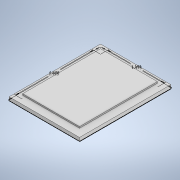
# Autodesk Inventor part: Valve Holder-3valve-withwirebox-lidforbox
Saved by Autodesk Inventor 2020 (Build 240168000, 168)
## iProperties
Created: 2022-02-08
Part Number: Valve Holder-3valve-withwirebox-lidforbox
Material: Generic
Document SubType Name: Modeling
Designer: Beaucage
Density: 1 g/cm^3
Appearance: Default
Author: Beaucage
Autodesk Inventor part; units mm, degrees
ref_plane "YZ Plane" through (0, 0, 0) normal (1, 0, 0) x (0, 1, 0)
ref_plane "XZ Plane" through (0, 0, 0) normal (0, 1, 0) x (-1, 0, 0)
ref_plane "XY Plane" through (0, 0, 0) normal (0, 0, 1) x (1, 0, 0)
sketch "Sketch1" plane through (0, 0, 0) normal (0, 1, 0) x (-1, 0, 0)
  line L0 (0, 0) -> (37.465, 0)
  line L1 (37.465, 0) -> (37.465, -48.641)
  line L2 (37.465, -48.641) -> (0, -48.641)
  line L3 (0, -48.641) -> (0, 0)
  line L4 (4.2291, -4.2291) -> (34.5059, -4.2291)
  line L5 (34.5059, -4.2291) -> (34.5059, -45.6819)
  line L6 (34.5059, -45.6819) -> (4.2291, -45.6819)
  line L7 (4.2291, -45.6819) -> (4.2291, -4.2291)
  line L8 (4.2291, -4.2291) -> (34.5059, -45.6819) construction
  line L9 (34.5059, -4.2291) -> (4.2291, -45.6819) construction
  point P0 (19.3675, -24.9555)
  dimension "d0" = 37.465
  dimension "d1" = 48.641
  dimension "d2" = 30.2768
  dimension "d3" = 41.4528
  constraints: 20 end point, 4 parallel, 2 horizontal, 2 midpoint, 2 perpendicular
  measures "d0" distance of L1.end L2.end
  measures "d1" distance of L0.end L1.end
  measures "d2" distance of L5.end L6.end
  measures "d3" distance of L4.end L5.end
extrude "Extrusion1" add sketch "Sketch1" along normal blind 2.54 contours L4 L5 L6 L7
extrude "Extrusion2" add sketch "Sketch1" along normal blind 1.778
body "Solid1"
